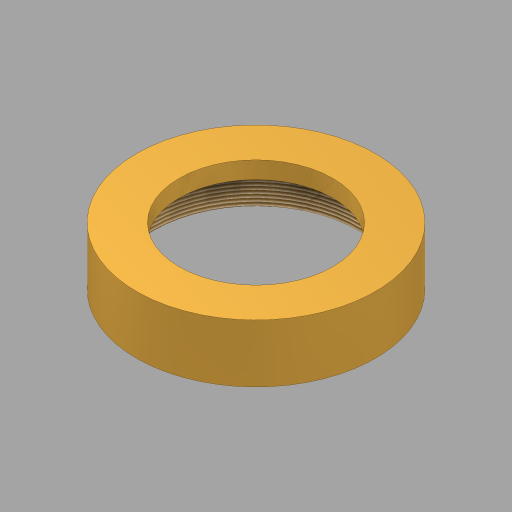
# Autodesk Inventor part: nut
Saved by Autodesk Inventor 2024 (Build 280153020, 153B)
## iProperties
Created: 2023-11-04
Part Number: nut
Material: Brass, Soft Yellow
Document SubType Name: Modeling
Designer: schanen
Density: 8.47 g/cm^3
Appearance: Brass - Satin
Mass: 201.04 g
Surface Area: 112.92 cm^2
Volume: 23.7355 cm^3
Author: schanen
Autodesk Inventor part; units mm, degrees
ref_plane "YZ Plane" through (0, 0, 0) normal (1, 0, 0) x (0, 1, 0)
ref_plane "XZ Plane" through (0, 0, 0) normal (0, 1, 0) x (-1, 0, 0)
ref_plane "XY Plane" through (0, 0, 0) normal (0, 0, 1) x (1, 0, 0)
sketch "Sketch1" plane through (0, 0, 0) normal (0, 0, 1) x (1, 0, 0)
  line L0 (-30, 0) -> (-30, 12)
  line L1 (-30, 12) -> (-22.5, 12)
  line L2 (-22.5, 12) -> (-22.5, 17)
  line L3 (-22.5, 17) -> (-35, 17)
  line L4 (-35, 17) -> (-35, 0)
  line L5 (-35, 0) -> (-30, 0)
  line L6 (0, -3.4) -> (0, 20.4) projected
  point P0 (0, 0)
  dimension "d1" = 30
  dimension "d2" = 12
  dimension "d3" = 5
  dimension "d4" = 22.5
  dimension "d5" = 5
  constraints: 12 end point, 5 perpendicular, 1 horizontal alignment, 1 vertical
  measures "d1" distance from line of point (0, 0) L0
  measures "d2" distance of L0.start L0.end
  measures "d3" distance of L1.end L2.end
  measures "d4" distance from line of point (0, 0) L2
  measures "d5" distance of L4.end L0.start
revolve "Revolution1" add sketch "Sketch1" angle 360 about axis through (0, -10, 0) along (0, 1, 0)
thread "Thread1" size "M60x1" class "6H" standard "ANSI Metric M Profile" full length
equation "\"d1\" = neck_thread_dia"
equation "\"d2\" = neck_thread_len"
equation "\"d4\" = 0.5 * oring_id"
equation "\"neck_thread_len\" = 12"
equation "\"neck_thread_dia\" = 30"
equation "\"oring_id\" = 45"
body "Solid1"
